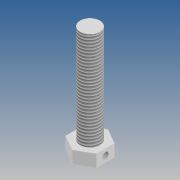
# Autodesk Inventor part: KB33-046-002-002 - Втулка
Saved by Autodesk Inventor 2020 (Build 240168000, 168)
## iProperties
Created: 2021-06-25
Part Number: KB33-046-002-002 - Втулка
Material: Типовые
Document SubType Name: Modeling
Designer: Петров Иван
Mass: 8.65083 g
Surface Area: 37.0496 cm^2
Volume: 8.65083 cm^3
Density: 1 g/cm^3
Appearance: По умолчанию
Author: Петров Иван
Autodesk Inventor part; units mm, degrees
ref_plane "YZ Plane" through (0, 0, 0) normal (1, 0, 0) x (0, 1, 0)
ref_plane "XZ Plane" through (0, 0, 0) normal (0, 1, 0) x (-1, 0, 0)
ref_plane "XY Plane" through (0, 0, 0) normal (0, 0, 1) x (1, 0, 0)
sketch "Эскиз1" plane through (0, 0, 0) normal (0, 1, 0) x (-1, 0, 0)
  circle A0 centre (0, 0) radius 6
  dimension "d0" = 12
  constraints: 1 centre point, 1 coincident
  measures "d0" diameter of A0
extrude "Выдавливание1" add sketch "Эскиз1" along normal blind 60
thread "Резьба1" size "M12x1.75" class "6g" standard "ANSI Metric M Profile" full length
sketch "Эскиз2" plane through (0, 0, 0) normal (0, -1, 0) x (1, 0, 0)
  line L0 (9.5, 5.4848) -> (9.5, -5.4848)
  line L1 (9.5, -5.4848) -> (0, -10.9697)
  line L2 (0, -10.9697) -> (-9.5, -5.4848)
  line L3 (-9.5, -5.4848) -> (-9.5, 5.4848)
  line L4 (-9.5, 5.4848) -> (0, 10.9697)
  line L5 (0, 10.9697) -> (9.5, 5.4848)
  line L6 (0, -15.3575) -> (0, 15.3575) construction
  point P0 (0, 0)
  point P1 (0, 0)
  dimension "d5" = 19
  constraints: 12 end point, 1 coincident, 1 parallel, 13 other
  measures "d5" distance between parallel lines of L3 L0
extrude "Выдавливание2" add sketch "Эскиз2" along normal blind 7.5
sketch "Эскиз3" plane through (0, -7.5, 0) normal (0, -1, 0) x (1, 0, 0)
  circle A0 centre (0, 0) radius 3
  dimension "d8" = 6
  constraints: 1 centre point, 1 coincident
  measures "d8" diameter of A0
extrude "Выдавливание3" cut sketch "Эскиз3" against normal blind 14
sketch "Эскиз4" plane through (9.5, 0, 5.4848) normal (1, 0, 0) x (0, 0, -1)
  circle A0 centre (5.4848, -3.75) radius 2
  line L0 (10.9697, -7.5) -> (0, -7.5) projected
  point P0 (5.4848, 0)
  dimension "d11" = 4
  dimension "d12" = 3.75
  constraints: 1 centre point
  measures "d11" diameter of A0
  measures "d12" distance from line of L0 A0.centre
extrude "Выдавливание4" cut sketch "Эскиз4" against normal blind 8.5
thread "Резьба2" size "M4x0.7" class "6H" standard "ANSI Metric M Profile" full length
